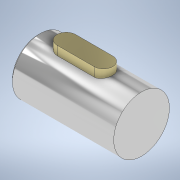
# Autodesk Inventor part: input shaft nmrv-40
Saved by Autodesk Inventor 2020 (Build 240168000, 168)
## iProperties
Created: 2020-08-01
Part Number: input shaft nmrv-40
Material: Generic
Document SubType Name: Modeling
Designer: Vikki
Density: 1 g/cm^3
Appearance: Chrome - Polished
Author: Vikki
Autodesk Inventor part; units mm, degrees
ref_plane "YZ Plane" through (0, 0, 0) normal (1, 0, 0) x (0, 1, 0)
ref_plane "XY Plane" through (0, 0, 0) normal (0, 0, 1) x (1, 0, 0)
sketch "Sketch1" plane through (0, 0, 0) normal (1, 0, 0) x (0, 1, 0)
  circle A0 centre (0, 0) radius 6
  dimension "d0" = 12
  constraints: 3 coincident, 1 centre point
  measures "d0" diameter of A0
extrude "Extrusion1" add sketch "Sketch1" along normal blind 22.2
ref_plane "Work Plane1" through (0, 6, 0) normal (0, 1, 0) x (-1, 0, 0)
sketch "Sketch2" plane through (0, 6, 0) normal (0, 1, 0) x (-1, 0, 0)
  line L0 (0, 6) -> (0, -6) projected
  line L1 (-6, 2) -> (-14, 2)
  line L2 (-16, 0) -> (-16, 0)
  line L3 (-14, -2) -> (-6, -2)
  line L4 (-4, 0) -> (-4, 0)
  arc A0 (-4, 0) -> (-6, 2) centre (-6, 0) ccw
  arc A1 (-6, -2) -> (-4, 0) centre (-6, 0) ccw
  arc A2 (-16, 0) -> (-14, -2) centre (-14, 0) ccw
  arc A3 (-14, 2) -> (-16, 0) centre (-14, 0) ccw
  point P0 (0, 0)
  point P1 (-16, -2)
  point P2 (-16, 2)
  point P3 (0, 0)
  point P4 (-16, 0)
  dimension "d3" = 4
  dimension "d4" = 2
  dimension "d5" = 6
  dimension "d6" = 8
  constraints: 8 end point, 8 point on circle, 8 tangent, 4 centre point, 4 point on line, 3 equal radius, 2 parallel, 1 horizontal, 1 horizontal alignment, 1 midpoint, 1 perpendicular
  measures "d3" distance of point (-16, 2) point (-16, -2)
  measures "d4" radius of A0
  measures "d5" distance from line of L0 A0.centre
  measures "d6" distance of A0.centre A2.centre
extrude "Extrusion2" add sketch "Sketch2" along normal blind 1.6 and the other way blind 1
chamfer "Chamfer1" distance 0.4 angle 45 1 edges at (0, -6, 0)
body "Solid1"
